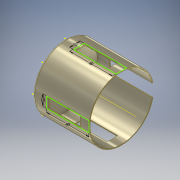
# Autodesk Inventor part: uMetal Can Backside
Saved by Autodesk Inventor 2017.3 (Build 213256000, 256)
## iProperties
Created: 2017-02-08
Part Number: uMetal Can Backside
Material: Generic
Document SubType Name: Modeling
Designer: Mac
Density: 1 g/cm^3
Appearance: Nickel
Author: Mac
Autodesk Inventor part; units mm, degrees
ref_plane "YZ Plane" through (0, 0, 0) normal (1, 0, 0) x (0, 1, 0)
sketch "Sketch1" plane through (0, 0, 0) normal (1, 0, 0) x (0, 1, 0)
  circle A0 centre (0, 0) radius 30.3
  dimension "d0" = 60.6
  constraints: 1 centre point, 1 coincident
  measures "d0" diameter of A0
extrude "Extrusion1" add sketch "Sketch1" along normal blind 53.1
sketch "Sketch2" plane through (53.1, 0, 0) normal (1, 0, 0) x (0, 0, -1)
  circle A0 centre (0, 0) radius 29.5
  dimension "d3" = 59
  constraints: 1 centre point, 1 coincident
  measures "d3" diameter of A0
extrude "Extrusion2" cut sketch "Sketch2" against normal blind 52.3
fillet "Fillet1" radius 2 1 edges at (0, -30.3, 0)
sketch "Sketch3" plane through (0.8, 0, 0) normal (1, 0, 0) x (0, 0, -1)
  circle A0 centre (0, 0) radius 1.5
  dimension "d7" = 3
  constraints: 1 centre point, 1 coincident
  measures "d7" diameter of A0
extrude "Extrusion3" [suppressed]
ref_plane "Work Plane2" through (0, -30.3, 0) normal (0, -1, 0) x (1, 0, 0)
ref_plane "Work Plane1" through (0, 30.3, 0) normal (0, 1, 0) x (-1, 0, 0)
ref_plane "Work Plane4" through (0, 0, -30.3) normal (0, 0, -1) x (-1, 0, 0)
ref_plane "Work Plane3" through (0, 0, 30.3) normal (0, 0, 1) x (1, 0, 0)
sketch "Sketch4" plane through (0, 30.3, 0) normal (0, 1, 0) x (-1, 0, 0)
  line L0 (-12.9, 5) -> (-52.9, 5)
  line L1 (-52.9, 5) -> (-52.9, -5)
  line L2 (-52.9, -5) -> (-12.9, -5)
  line L3 (-12.9, -5) -> (-12.9, 5)
  line L4 (-52.9, -5) -> (-68.7786, -5)
  line L5 (-68.7786, -5) -> (-68.7786, 5)
  line L6 (-68.7786, 5) -> (-52.9, 5)
  line L7 (-52.9, 5) -> (-52.9, -5)
  point P0 (0, 0)
  point P1 (-32.9, 0)
  dimension "d14" = 40
  dimension "d15" = 10
  constraints: 16 end point, 4 parallel, 2 horizontal, 2 perpendicular
  measures "d14" distance of L2.end L1.end
  measures "d15" distance of L1.end L0.end
sketch "Sketch6" plane through (0, 0, -30.3) normal (0, 0, -1) x (-1, 0, 0)
  line L0 (-14.5434, 5) -> (-44.5434, 5)
  line L1 (-44.5434, 5) -> (-44.5434, -5)
  line L2 (-44.5434, -5) -> (-14.5434, -5)
  line L3 (-14.5434, -5) -> (-14.5434, 5)
  point P0 (0, 0)
  dimension "d16" = 30
  dimension "d17" = 10
  constraints: 8 end point, 2 parallel, 1 horizontal, 1 perpendicular
  measures "d16" distance of L2.end L2.start
  measures "d17" distance of L2.start L0.end
sketch "Sketch7" plane through (0, 0, 30.3) normal (0, 0, 1) x (1, 0, 0)
  line L0 (52.8787, 5) -> (12.8787, 5)
  line L1 (12.8787, 5) -> (12.8787, -5)
  line L2 (12.8787, -5) -> (52.8787, -5)
  line L3 (52.8787, -5) -> (52.8787, 5)
  point P0 (0, 0)
  dimension "d18" = 40
  dimension "d19" = 10
  constraints: 8 end point, 2 parallel, 1 horizontal, 1 perpendicular
  measures "d18" distance of L2.end L2.start
  measures "d19" distance of L2.start L0.end
sketch "Sketch8" plane through (0, -30.3, 0) normal (0, -1, 0) x (1, 0, 0)
  point P0 (0, 0)
sketch "Sketch9" plane through (0, -30.3, 0) normal (0, -1, 0) x (1, 0, 0)
  point P0 (0, 0)
sketch "Sketch10" plane through (0, -30.3, 0) normal (0, -1, 0) x (1, 0, 0)
  line L0 (12.8787, -5) -> (52.8787, -5)
  line L1 (52.8787, -5) -> (52.8787, 5)
  line L2 (52.8787, 5) -> (12.8787, 5)
  line L3 (12.8787, 5) -> (12.8787, -5)
  point P0 (0, 0)
  dimension "d20" = 40
  dimension "d21" = 10
  constraints: 8 end point, 2 parallel, 1 horizontal, 1 perpendicular
  measures "d20" distance of L0.end L0.start
  measures "d21" distance of L0.start L2.end
extrude "Extrusion6" cut sketch "Sketch6" against normal blind 5
extrude "Extrusion7" cut sketch "Sketch4" against normal blind 5
ref_plane "Work Plane5" through (53.1, 0, 0) normal (0, -0.7071068, -0.7071068) x (1, 0, 0)
ref_plane "Work Plane6" through (53.1, 0, 0) normal (0, 0.7071068, -0.7071068) x (1, 0, 0)
ref_plane "Work Plane7" through (53.1, -21.4253, 21.4253) normal (0, -0.7071068, 0.7071068) x (1, 0, 0)
ref_plane "Work Plane8" through (53.1, 21.4253, -21.4253) normal (0, 0.7071068, -0.7071068) x (1, 0, 0)
ref_plane "Work Plane9" through (53.1, 21.4253, 21.4253) normal (0, 0.7071068, 0.7071068) x (-1, 0, 0)
ref_plane "Work Plane10" through (53.1, -21.4253, -21.4253) normal (0, -0.7071068, -0.7071068) x (1, 0, 0)
sketch "Sketch11" plane through (53.1, -21.4253, -21.4253) normal (0, -0.7071068, -0.7071068) x (1, 0, 0)
  point P0 (-53.1, 0)
sketch "Sketch12" plane through (53.1, 21.4253, -21.4253) normal (0, 0.7071068, -0.7071068) x (1, 0, 0)
  point P0 (-53.1, 0)
sketch "Sketch13" plane through (53.1, -21.4253, 21.4253) normal (0, -0.7071068, 0.7071068) x (1, 0, 0)
  point P0 (-53.1, 0)
sketch "Sketch15" plane through (0, 0, 0) normal (-1, 0, 0) x (0, 0, 1)
  point P0 (0, 0)
  point P1 (0, 10.7)
  point P2 (9.2665, -5.35)
  point P3 (-9.2665, -5.35)
hole "Hole6" [suppressed]
sketch "Sketch17" plane through (12.9, 29.8846, -5) normal (0, 0, 1) x (1, 0, 0)
  line L0 (0, 0.4154) -> (0, 0) projected
  line L1 (0, 0) -> (56.3299, 0)
  line L2 (56.3299, 0) -> (56.3299, -2.903)
  line L3 (56.3299, -2.903) -> (0, -2.903)
  line L4 (0, -2.903) -> (0, 0)
  point P0 (-12.9, -29.8846)
  constraints: 8 end point, 2 parallel, 1 horizontal, 1 perpendicular
extrude "Extrusion8" cut sketch "Sketch17" against normal blind 1
sketch "Sketch18" plane through (53.1, 29.8846, 5) normal (0, 0, -1) x (-1, 0, 0)
  line L0 (0, 0) -> (40.2, 0) projected
  line L1 (40.2, 0) -> (-20.2258, 0)
  line L2 (-20.2258, 0) -> (-20.2258, -6.4784)
  line L3 (-20.2258, -6.4784) -> (40.2, -6.4784)
  line L4 (40.2, -6.4784) -> (40.2, 0)
  point P0 (53.1, -29.8846)
  constraints: 8 end point, 2 parallel, 1 horizontal, 1 perpendicular
extrude "Extrusion9" cut sketch "Sketch18" against normal blind 1
pattern_circular "Circular Pattern1" count 3 over 180 about axis through (53.1, 0, 0) along (-1, 0, 0) of "Extrusion6"
body "Solid1"
